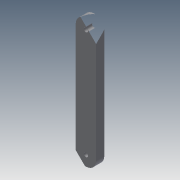
# Autodesk Inventor part: drivelever
Saved by Autodesk Inventor 2015 (Build 190159000, 159)
## iProperties
Created: 2014-08-31
Part Number: drivelever
Material: Generic
Document SubType Name: Modeling
Designer: shohei
Density: 1 g/cm^3
Appearance: Default
Author: shohei
Autodesk Inventor part; units mm, degrees
ref_plane "YZ Plane" through (0, 0, 0) normal (1, 0, 0) x (0, 1, 0)
ref_plane "XZ Plane" through (0, 0, 0) normal (0, 1, 0) x (-1, 0, 0)
ref_plane "XY Plane" through (0, 0, 0) normal (0, 0, 1) x (1, 0, 0)
sketch "Sketch1" plane through (0, 0, 0) normal (0, 1, 0) x (-1, 0, 0)
  arc A0 (-25, 0) -> (25, 0) centre (0, 0) ccw
  arc A1 (25, 285) -> (-25, 285) centre (0, 285) ccw
  line L0 (25, 285) -> (25, 0)
  line L1 (-25, 0) -> (-25, 285)
  circle A2 centre (0, 285) radius 5
  circle A3 centre (0, 0) radius 5
  dimension "d0" = 50
  dimension "d1" = 50
  dimension "d2" = 10
  dimension "d3" = 10
  dimension "d6" = 285
  constraints: 4 centre point, 4 end point, 4 point on circle, 3 coincident, 3 tangent
  measures "d0" diameter of A0
  measures "d1" diameter of A1
  measures "d2" diameter of A2
  measures "d3" diameter of A3
  measures "d6" distance of L0.start L0.end
extrude "Extrusion1" add sketch "Sketch1" along normal blind 20
equation "\"d6\" = 0.95 * pD"
equation "\"pD\" = 300"
body "Solid1"
